Autodesk Fusion 360 part; units mm, degrees
note: some values were not read from the file. Chosen so that the rebuilt part matches the saved one: which bodies a step acts on.
(part 2 of 2)
extrude "Extrude1''''''''''''''''''''''''''''''" add sketch "Motor_Pulley_Sketch" along normal blind 6 from surface at 16 separate body makes body 36 in component "Motor_Pulley"
sketch "Tension_Slot_-11_16" plane through (0, 0, 0) normal (0, 0, 1) x (1, 0, 0) in component "Base_Plate_Al"
  line L0 (-12.7, 13) -> (-9.3, 13)
  line L1 (-9.3, 13) -> (-9.3, 19)
  line L2 (-9.3, 19) -> (-12.7, 19)
  line L3 (-12.7, 19) -> (-12.7, 13)
extrude "Extrude15'" cut sketch "Tension_Slot_-11_16" along normal blind 6 from surface at 1 bodies 1 in component "Base_Plate_Al"
sketch "Tension_Slot_11_16" plane through (0, 0, 0) normal (0, 0, 1) x (1, 0, 0) in component "Base_Plate_Al"
  line L0 (9.3, 13) -> (12.7, 13)
  line L1 (12.7, 13) -> (12.7, 19)
  line L2 (12.7, 19) -> (9.3, 19)
  line L3 (9.3, 19) -> (9.3, 13)
extrude "Extrude16" cut sketch "Tension_Slot_11_16" along normal blind 6 from surface at 1 bodies 1 in component "Base_Plate_Al"
sketch "Tension_Slot_-11_37" plane through (0, 0, 0) normal (0, 0, 1) x (1, 0, 0) in component "Base_Plate_Al"
  line L0 (-12.7, 34) -> (-9.3, 34)
  line L1 (-9.3, 34) -> (-9.3, 40)
  line L2 (-9.3, 40) -> (-12.7, 40)
  line L3 (-12.7, 40) -> (-12.7, 34)
extrude "Extrude17" cut sketch "Tension_Slot_-11_37" along normal blind 6 from surface at 1 bodies 1 in component "Base_Plate_Al"
sketch "Tension_Slot_11_37" plane through (0, 0, 0) normal (0, 0, 1) x (1, 0, 0) in component "Base_Plate_Al"
  line L0 (9.3, 34) -> (12.7, 34)
  line L1 (12.7, 34) -> (12.7, 40)
  line L2 (12.7, 40) -> (9.3, 40)
  line L3 (9.3, 40) -> (9.3, 34)
extrude "Extrude18" cut sketch "Tension_Slot_11_37" along normal blind 6 from surface at 1 bodies 1 in component "Base_Plate_Al"
sketch "Shaft_Bore" plane through (0, 0, 0) normal (1, 0, 0) x (0, 0, -1) in component "Weapon_Pulley"
  circle A0 centre (-38.5, 75) radius 2
extrude "Extrude2''''''''''''''''''''''''" cut sketch "Shaft_Bore" along normal mid plane 400 bodies 35 in component "Weapon_Pulley"
sketch "Shaft_Bore (2)" plane through (0, 0, 0) normal (1, 0, 0) x (0, 0, -1) in component "Left_Support"
  circle A0 centre (-38.5, 75) radius 2
extrude "Extrude2'''''''''''''''''''''''''" cut sketch "Shaft_Bore (2)" along normal mid plane 400 bodies 15 in component "Left_Support"
sketch "Shaft_Bore (3)" plane through (0, 0, 0) normal (1, 0, 0) x (0, 0, -1) in component "Right_Support"
  circle A0 centre (-38.5, 75) radius 2
extrude "Extrude2''''''''''''''''''''''''''" cut sketch "Shaft_Bore (3)" along normal mid plane 400 bodies 16 in component "Right_Support"
sketch "Shaft_Bore (4)" plane through (0, 0, 0) normal (1, 0, 0) x (0, 0, -1) in component "Motor_Pulley"
  circle A0 centre (-38.5, 25.75) radius 1.585
extrude "Extrude2'''''''''''''''''''''''''''" cut sketch "Shaft_Bore (4)" along normal mid plane 400 bodies 36 in component "Motor_Pulley"
sketch "Wedge_HoldDown_Clear" plane through (0, 0, 0) normal (0, 0, 1) x (1, 0, 0) in component "Front_Wedge_L"
  circle A0 centre (-73, 80) radius 1.7
  circle A1 centre (-50, 50) radius 1.7
extrude "Extrude5'''''''" cut sketch "Wedge_HoldDown_Clear" along normal blind 6 from surface at 4 bodies 12 in component "Front_Wedge_L"
sketch "Wedge_HoldDown_Clear (2)" plane through (0, 0, 0) normal (0, 0, 1) x (1, 0, 0) in component "Front_Wedge_R"
  circle A0 centre (50, 50) radius 1.7
  circle A1 centre (73, 80) radius 1.7
extrude "Extrude5''''''''" cut sketch "Wedge_HoldDown_Clear (2)" along normal blind 6 from surface at 4 bodies 13 in component "Front_Wedge_R"
sketch "ESC_Tekko32_Sketch" plane through (0, 0, 0) normal (0, 0, 1) x (1, 0, 0) in component "ESC_Tekko32"
  line L0 (17.85, 19.35) -> (52.15, 19.35)
  line L1 (52.15, 19.35) -> (52.15, 36.65)
  line L2 (52.15, 36.65) -> (17.85, 36.65)
  line L3 (17.85, 36.65) -> (17.85, 19.35)
extrude "Extrude1'''''''''''''''''''''''''''''''" add sketch "ESC_Tekko32_Sketch" along normal blind 4.5 from surface at 7 separate body makes body 37 in component "ESC_Tekko32"
sketch "Holder_ESC_Tekko32_Sketch" plane through (0, 0, 0) normal (0, 0, 1) x (1, 0, 0) in component "Holder_ESC_Tekko32"
  line L0 (16.05, 17.55) -> (53.95, 17.55)
  line L1 (53.95, 17.55) -> (53.95, 38.45)
  line L2 (53.95, 38.45) -> (16.05, 38.45)
  line L3 (16.05, 38.45) -> (16.05, 17.55)
extrude "Extrude1''''''''''''''''''''''''''''''''" add sketch "Holder_ESC_Tekko32_Sketch" along normal blind 5.5 from surface at 5 separate body makes body 38 in component "Holder_ESC_Tekko32"
sketch "Holder_ESC_Tekko32_Pocket" plane through (0, 0, 0) normal (0, 0, 1) x (1, 0, 0) in component "Holder_ESC_Tekko32"
  line L0 (17.65, 19.15) -> (52.35, 19.15)
  line L1 (52.35, 19.15) -> (52.35, 36.85)
  line L2 (52.35, 36.85) -> (17.65, 36.85)
  line L3 (17.65, 36.85) -> (17.65, 19.15)
extrude "Extrude2''''''''''''''''''''''''''''" cut sketch "Holder_ESC_Tekko32_Pocket" along normal blind 60 from surface at 7 bodies 38 in component "Holder_ESC_Tekko32"
sketch "Holder_ESC_Tekko32_TieGroove" plane through (0, 0, 0) normal (0, 0, 1) x (1, 0, 0) in component "Holder_ESC_Tekko32"
  line L0 (33, 16.55) -> (37, 16.55)
  line L1 (37, 16.55) -> (37, 39.45)
  line L2 (37, 39.45) -> (33, 39.45)
  line L3 (33, 39.45) -> (33, 16.55)
extrude "Extrude3''''''''''''''''" cut sketch "Holder_ESC_Tekko32_TieGroove" along normal blind 2.2 from surface at 4 bodies 38 in component "Holder_ESC_Tekko32"
sketch "Holder_ESC_Tekko32_FloorHoles" plane through (0, 0, 0) normal (0, 0, 1) x (1, 0, 0) in component "Holder_ESC_Tekko32"
  circle A0 centre (21.85, 28) radius 1.7
  circle A1 centre (48.15, 28) radius 1.7
extrude "Extrude4''''''''''''" cut sketch "Holder_ESC_Tekko32_FloorHoles" along normal blind 4 from surface at 4 bodies 38 in component "Holder_ESC_Tekko32"
sketch "Holder_ESC_Tekko32_PlateHoles" plane through (0, 0, 0) normal (0, 0, 1) x (1, 0, 0) in component "Base_Plate_Al"
  circle A0 centre (21.85, 28) radius 1.25
  circle A1 centre (48.15, 28) radius 1.25
extrude "Extrude23" cut sketch "Holder_ESC_Tekko32_PlateHoles" along normal blind 6 from surface at 1 bodies 1 in component "Base_Plate_Al"
sketch "Rx_ER6_Sketch" plane through (0, 0, 0) normal (0, 0, 1) x (1, 0, 0) in component "Rx_ER6"
  line L0 (-64.5, -84.5) -> (-39.5, -84.5)
  line L1 (-39.5, -84.5) -> (-39.5, -41.5)
  line L2 (-39.5, -41.5) -> (-64.5, -41.5)
  line L3 (-64.5, -41.5) -> (-64.5, -84.5)
extrude "Extrude1'''''''''''''''''''''''''''''''''" add sketch "Rx_ER6_Sketch" along normal blind 15 from surface at 7 separate body makes body 39 in component "Rx_ER6"
sketch "Holder_Rx_ER6_Sketch" plane through (0, 0, 0) normal (0, 0, 1) x (1, 0, 0) in component "Holder_Rx_ER6"
  line L0 (-66.3, -86.3) -> (-37.7, -86.3)
  line L1 (-37.7, -86.3) -> (-37.7, -39.7)
  line L2 (-37.7, -39.7) -> (-66.3, -39.7)
  line L3 (-66.3, -39.7) -> (-66.3, -86.3)
extrude "Extrude1''''''''''''''''''''''''''''''''''" add sketch "Holder_Rx_ER6_Sketch" along normal blind 16 from surface at 5 separate body makes body 40 in component "Holder_Rx_ER6"
sketch "Holder_Rx_ER6_Pocket" plane through (0, 0, 0) normal (0, 0, 1) x (1, 0, 0) in component "Holder_Rx_ER6"
  line L0 (-64.7, -84.7) -> (-39.3, -84.7)
  line L1 (-39.3, -84.7) -> (-39.3, -41.3)
  line L2 (-39.3, -41.3) -> (-64.7, -41.3)
  line L3 (-64.7, -41.3) -> (-64.7, -84.7)
extrude "Extrude2'''''''''''''''''''''''''''''" cut sketch "Holder_Rx_ER6_Pocket" along normal blind 60 from surface at 7 bodies 40 in component "Holder_Rx_ER6"
sketch "Holder_Rx_ER6_TieGroove" plane through (0, 0, 0) normal (0, 0, 1) x (1, 0, 0) in component "Holder_Rx_ER6"
  line L0 (-67.3, -65) -> (-36.7, -65)
  line L1 (-36.7, -65) -> (-36.7, -61)
  line L2 (-36.7, -61) -> (-67.3, -61)
  line L3 (-67.3, -61) -> (-67.3, -65)
extrude "Extrude3'''''''''''''''''" cut sketch "Holder_Rx_ER6_TieGroove" along normal blind 2.2 from surface at 4 bodies 40 in component "Holder_Rx_ER6"
sketch "Holder_Rx_ER6_FloorHoles" plane through (0, 0, 0) normal (0, 0, 1) x (1, 0, 0) in component "Holder_Rx_ER6"
  circle A0 centre (-52, -80.5) radius 1.7
  circle A1 centre (-52, -45.5) radius 1.7
extrude "Extrude4'''''''''''''" cut sketch "Holder_Rx_ER6_FloorHoles" along normal blind 4 from surface at 4 bodies 40 in component "Holder_Rx_ER6"
sketch "Holder_Rx_ER6_PlateHoles" plane through (0, 0, 0) normal (0, 0, 1) x (1, 0, 0) in component "Base_Plate_Al"
  circle A0 centre (-52, -80.5) radius 1.25
  circle A1 centre (-52, -45.5) radius 1.25
extrude "Extrude24" cut sketch "Holder_Rx_ER6_PlateHoles" along normal blind 6 from surface at 1 bodies 1 in component "Base_Plate_Al"
sketch "UBEC_5A_Sketch" plane through (0, 0, 0) normal (0, 0, 1) x (1, 0, 0) in component "UBEC_5A"
  line L0 (57.5, -76) -> (74.5, -76)
  line L1 (74.5, -76) -> (74.5, -26)
  line L2 (74.5, -26) -> (57.5, -26)
  line L3 (57.5, -26) -> (57.5, -76)
extrude "Extrude1'''''''''''''''''''''''''''''''''''" add sketch "UBEC_5A_Sketch" along normal blind 10 from surface at 7 separate body makes body 41 in component "UBEC_5A"
sketch "Holder_UBEC_5A_Sketch" plane through (0, 0, 0) normal (0, 0, 1) x (1, 0, 0) in component "Holder_UBEC_5A"
  line L0 (55.7, -77.8) -> (76.3, -77.8)
  line L1 (76.3, -77.8) -> (76.3, -24.2)
  line L2 (76.3, -24.2) -> (55.7, -24.2)
  line L3 (55.7, -24.2) -> (55.7, -77.8)
extrude "Extrude1''''''''''''''''''''''''''''''''''''" add sketch "Holder_UBEC_5A_Sketch" along normal blind 11 from surface at 5 separate body makes body 42 in component "Holder_UBEC_5A"
sketch "Holder_UBEC_5A_Pocket" plane through (0, 0, 0) normal (0, 0, 1) x (1, 0, 0) in component "Holder_UBEC_5A"
  line L0 (57.3, -76.2) -> (74.7, -76.2)
  line L1 (74.7, -76.2) -> (74.7, -25.8)
  line L2 (74.7, -25.8) -> (57.3, -25.8)
  line L3 (57.3, -25.8) -> (57.3, -76.2)
extrude "Extrude2''''''''''''''''''''''''''''''" cut sketch "Holder_UBEC_5A_Pocket" along normal blind 60 from surface at 7 bodies 42 in component "Holder_UBEC_5A"
sketch "Holder_UBEC_5A_TieGroove" plane through (0, 0, 0) normal (0, 0, 1) x (1, 0, 0) in component "Holder_UBEC_5A"
  line L0 (54.7, -53) -> (77.3, -53)
  line L1 (77.3, -53) -> (77.3, -49)
  line L2 (77.3, -49) -> (54.7, -49)
  line L3 (54.7, -49) -> (54.7, -53)
extrude "Extrude3''''''''''''''''''" cut sketch "Holder_UBEC_5A_TieGroove" along normal blind 2.2 from surface at 4 bodies 42 in component "Holder_UBEC_5A"
sketch "Holder_UBEC_5A_FloorHoles" plane through (0, 0, 0) normal (0, 0, 1) x (1, 0, 0) in component "Holder_UBEC_5A"
  circle A0 centre (66, -72) radius 1.7
  circle A1 centre (66, -30) radius 1.7
extrude "Extrude4''''''''''''''" cut sketch "Holder_UBEC_5A_FloorHoles" along normal blind 4 from surface at 4 bodies 42 in component "Holder_UBEC_5A"
sketch "Holder_UBEC_5A_PlateHoles" plane through (0, 0, 0) normal (0, 0, 1) x (1, 0, 0) in component "Base_Plate_Al"
  circle A0 centre (66, -72) radius 1.25
  circle A1 centre (66, -30) radius 1.25
extrude "Extrude25" cut sketch "Holder_UBEC_5A_PlateHoles" along normal blind 6 from surface at 1 bodies 1 in component "Base_Plate_Al"
sketch "DRV8874_A_Sketch" plane through (0, 0, 0) normal (0, 0, 1) x (1, 0, 0) in component "DRV8874_A"
  line L0 (-34.9, -81.6) -> (-17.1, -81.6)
  line L1 (-17.1, -81.6) -> (-17.1, -66.4)
  line L2 (-17.1, -66.4) -> (-34.9, -66.4)
  line L3 (-34.9, -66.4) -> (-34.9, -81.6)
extrude "Extrude1'''''''''''''''''''''''''''''''''''''" add sketch "DRV8874_A_Sketch" along normal blind 3 from surface at 7 separate body makes body 43 in component "DRV8874_A"
sketch "Holder_DRV8874_A_Sketch" plane through (0, 0, 0) normal (0, 0, 1) x (1, 0, 0) in component "Holder_DRV8874_A"
  line L0 (-36.7, -83.4) -> (-15.3, -83.4)
  line L1 (-15.3, -83.4) -> (-15.3, -64.6)
  line L2 (-15.3, -64.6) -> (-36.7, -64.6)
  line L3 (-36.7, -64.6) -> (-36.7, -83.4)
extrude "Extrude1''''''''''''''''''''''''''''''''''''''" add sketch "Holder_DRV8874_A_Sketch" along normal blind 4 from surface at 5 separate body makes body 44 in component "Holder_DRV8874_A"
sketch "Holder_DRV8874_A_Pocket" plane through (0, 0, 0) normal (0, 0, 1) x (1, 0, 0) in component "Holder_DRV8874_A"
  line L0 (-35.1, -81.8) -> (-16.9, -81.8)
  line L1 (-16.9, -81.8) -> (-16.9, -66.2)
  line L2 (-16.9, -66.2) -> (-35.1, -66.2)
  line L3 (-35.1, -66.2) -> (-35.1, -81.8)
extrude "Extrude2'''''''''''''''''''''''''''''''" cut sketch "Holder_DRV8874_A_Pocket" along normal blind 60 from surface at 7 bodies 44 in component "Holder_DRV8874_A"
sketch "Holder_DRV8874_A_TieGroove" plane through (0, 0, 0) normal (0, 0, 1) x (1, 0, 0) in component "Holder_DRV8874_A"
  line L0 (-28, -84.4) -> (-24, -84.4)
  line L1 (-24, -84.4) -> (-24, -63.6)
  line L2 (-24, -63.6) -> (-28, -63.6)
  line L3 (-28, -63.6) -> (-28, -84.4)
extrude "Extrude3'''''''''''''''''''" cut sketch "Holder_DRV8874_A_TieGroove" along normal blind 2.2 from surface at 4 bodies 44 in component "Holder_DRV8874_A"
sketch "Holder_DRV8874_A_FloorHoles" plane through (0, 0, 0) normal (0, 0, 1) x (1, 0, 0) in component "Holder_DRV8874_A"
  circle A0 centre (-31, -74) radius 1.7
  circle A1 centre (-21, -74) radius 1.7
extrude "Extrude4'''''''''''''''" cut sketch "Holder_DRV8874_A_FloorHoles" along normal blind 4 from surface at 4 bodies 44 in component "Holder_DRV8874_A"
sketch "Holder_DRV8874_A_PlateHoles" plane through (0, 0, 0) normal (0, 0, 1) x (1, 0, 0) in component "Base_Plate_Al"
  circle A0 centre (-31, -74) radius 1.25
  circle A1 centre (-21, -74) radius 1.25
extrude "Extrude26" cut sketch "Holder_DRV8874_A_PlateHoles" along normal blind 6 from surface at 1 bodies 1 in component "Base_Plate_Al"
sketch "DRV8874_B_Sketch" plane through (0, 0, 0) normal (0, 0, 1) x (1, 0, 0) in component "DRV8874_B"
  line L0 (-11.6, -83.9) -> (3.6, -83.9)
  line L1 (3.6, -83.9) -> (3.6, -66.1)
  line L2 (3.6, -66.1) -> (-11.6, -66.1)
  line L3 (-11.6, -66.1) -> (-11.6, -83.9)
extrude "Extrude1'''''''''''''''''''''''''''''''''''''''" add sketch "DRV8874_B_Sketch" along normal blind 3 from surface at 7 separate body makes body 45 in component "DRV8874_B"
sketch "Holder_DRV8874_B_Sketch" plane through (0, 0, 0) normal (0, 0, 1) x (1, 0, 0) in component "Holder_DRV8874_B"
  line L0 (-13.4, -85.7) -> (5.4, -85.7)
  line L1 (5.4, -85.7) -> (5.4, -64.3)
  line L2 (5.4, -64.3) -> (-13.4, -64.3)
  line L3 (-13.4, -64.3) -> (-13.4, -85.7)
extrude "Extrude1''''''''''''''''''''''''''''''''''''''''" add sketch "Holder_DRV8874_B_Sketch" along normal blind 4 from surface at 5 separate body makes body 46 in component "Holder_DRV8874_B"
sketch "Holder_DRV8874_B_Pocket" plane through (0, 0, 0) normal (0, 0, 1) x (1, 0, 0) in component "Holder_DRV8874_B"
  line L0 (-11.8, -84.1) -> (3.8, -84.1)
  line L1 (3.8, -84.1) -> (3.8, -65.9)
  line L2 (3.8, -65.9) -> (-11.8, -65.9)
  line L3 (-11.8, -65.9) -> (-11.8, -84.1)
extrude "Extrude2''''''''''''''''''''''''''''''''" cut sketch "Holder_DRV8874_B_Pocket" along normal blind 60 from surface at 7 bodies 46 in component "Holder_DRV8874_B"
sketch "Holder_DRV8874_B_TieGroove" plane through (0, 0, 0) normal (0, 0, 1) x (1, 0, 0) in component "Holder_DRV8874_B"
  line L0 (-14.4, -77) -> (6.4, -77)
  line L1 (6.4, -77) -> (6.4, -73)
  line L2 (6.4, -73) -> (-14.4, -73)
  line L3 (-14.4, -73) -> (-14.4, -77)
extrude "Extrude3''''''''''''''''''''" cut sketch "Holder_DRV8874_B_TieGroove" along normal blind 2.2 from surface at 4 bodies 46 in component "Holder_DRV8874_B"
sketch "Holder_DRV8874_B_FloorHoles" plane through (0, 0, 0) normal (0, 0, 1) x (1, 0, 0) in component "Holder_DRV8874_B"
  circle A0 centre (-4, -80) radius 1.7
  circle A1 centre (-4, -70) radius 1.7
extrude "Extrude4''''''''''''''''" cut sketch "Holder_DRV8874_B_FloorHoles" along normal blind 4 from surface at 4 bodies 46 in component "Holder_DRV8874_B"
sketch "Holder_DRV8874_B_PlateHoles" plane through (0, 0, 0) normal (0, 0, 1) x (1, 0, 0) in component "Base_Plate_Al"
  circle A0 centre (-4, -80) radius 1.25
  circle A1 centre (-4, -70) radius 1.25
extrude "Extrude27" cut sketch "Holder_DRV8874_B_PlateHoles" along normal blind 6 from surface at 1 bodies 1 in component "Base_Plate_Al"
sketch "ESP32_DevKit_Sketch" plane through (0, 0, 0) normal (0, 0, 1) x (1, 0, 0) in component "ESP32_DevKit"
  line L0 (-25.75, -52.15) -> (25.75, -52.15)
  line L1 (25.75, -52.15) -> (25.75, -23.85)
  line L2 (25.75, -23.85) -> (-25.75, -23.85)
  line L3 (-25.75, -23.85) -> (-25.75, -52.15)
extrude "Extrude1'''''''''''''''''''''''''''''''''''''''''" add sketch "ESP32_DevKit_Sketch" along normal blind 1.6 from surface at 25 separate body makes body 47 in component "ESP32_DevKit"
sketch "ESP32_Holes" plane through (0, 0, 0) normal (0, 0, 1) x (1, 0, 0) in component "ESP32_DevKit"
  circle A0 centre (-23.6, -49.7) radius 1.3
  circle A1 centre (-23.6, -26.3) radius 1.3
  circle A2 centre (23.6, -49.7) radius 1.3
  circle A3 centre (23.6, -26.3) radius 1.3
extrude "Extrude2'''''''''''''''''''''''''''''''''" cut sketch "ESP32_Holes" along normal blind 3.6 from surface at 24 bodies 47 in component "ESP32_DevKit"
sketch "ESP32_Module_Sketch" plane through (0, 0, 0) normal (0, 0, 1) x (1, 0, 0) in component "ESP32_DevKit"
  line L0 (-25.75, -47) -> (-0.25, -47)
  line L1 (-0.25, -47) -> (-0.25, -29)
  line L2 (-0.25, -29) -> (-25.75, -29)
  line L3 (-25.75, -29) -> (-25.75, -47)
extrude "Extrude3'''''''''''''''''''''" add sketch "ESP32_Module_Sketch" along normal blind 3.1 from surface at 26.6 separate body makes body 48 in component "ESP32_DevKit"
sketch "ESP32_Dupont_Keepout_A_Sketch" plane through (0, 0, 0) normal (0, 0, 1) x (1, 0, 0) in component "ESP32_DevKit"
  line L0 (-20.72, -51.97) -> (14.88, -51.97)
  line L1 (14.88, -51.97) -> (14.88, -49.43)
  line L2 (14.88, -49.43) -> (-20.72, -49.43)
  line L3 (-20.72, -49.43) -> (-20.72, -51.97)
extrude "Extrude4'''''''''''''''''" add sketch "ESP32_Dupont_Keepout_A_Sketch" along normal blind 16.5 from surface at 8.5 separate body makes body 49 in component "ESP32_DevKit"
sketch "ESP32_Dupont_Keepout_B_Sketch" plane through (0, 0, 0) normal (0, 0, 1) x (1, 0, 0) in component "ESP32_DevKit"
  line L0 (-20.72, -26.57) -> (14.88, -26.57)
  line L1 (14.88, -26.57) -> (14.88, -24.03)
  line L2 (14.88, -24.03) -> (-20.72, -24.03)
  line L3 (-20.72, -24.03) -> (-20.72, -26.57)
extrude "Extrude5'''''''''" add sketch "ESP32_Dupont_Keepout_B_Sketch" along normal blind 16.5 from surface at 8.5 separate body makes body 50 in component "ESP32_DevKit"
sketch "Holder_ESP32_Sketch" plane through (0, 0, 0) normal (0, 0, 1) x (1, 0, 0) in component "Holder_ESP32"
  line L0 (-27.75, -54.15) -> (27.75, -54.15)
  line L1 (27.75, -54.15) -> (27.75, -21.85)
  line L2 (27.75, -21.85) -> (-27.75, -21.85)
  line L3 (-27.75, -21.85) -> (-27.75, -54.15)
extrude "Extrude1''''''''''''''''''''''''''''''''''''''''''" add sketch "Holder_ESP32_Sketch" along normal blind 2 from surface at 5 separate body makes body 51 in component "Holder_ESP32"
sketch "Holder_ESP32_Posts" plane through (0, 0, 0) normal (0, 0, 1) x (1, 0, 0) in component "Holder_ESP32"
  circle A0 centre (-23.6, -49.7) radius 2.25
  circle A1 centre (-23.6, -26.3) radius 2.25
  circle A2 centre (23.6, -49.7) radius 2.25
  circle A3 centre (23.6, -26.3) radius 2.25
extrude "Extrude2''''''''''''''''''''''''''''''''''" add sketch "Holder_ESP32_Posts" along normal blind 18 from surface at 7 bodies 51 in component "Holder_ESP32"
sketch "Holder_ESP32_Window" plane through (0, 0, 0) normal (0, 0, 1) x (1, 0, 0) in component "Holder_ESP32"
  line L0 (-9, -47.15) -> (9, -47.15)
  line L1 (9, -47.15) -> (9, -28.85)
  line L2 (9, -28.85) -> (-9, -28.85)
  line L3 (-9, -28.85) -> (-9, -47.15)
extrude "Extrude3''''''''''''''''''''''" cut sketch "Holder_ESP32_Window" along normal blind 4 from surface at 4 bodies 51 in component "Holder_ESP32"
sketch "Holder_ESP32_PostPilots" plane through (0, 0, 0) normal (0, 0, 1) x (1, 0, 0) in component "Holder_ESP32"
  circle A0 centre (-23.6, -49.7) radius 0.8
  circle A1 centre (-23.6, -26.3) radius 0.8
  circle A2 centre (23.6, -49.7) radius 0.8
  circle A3 centre (23.6, -26.3) radius 0.8
extrude "Extrude4''''''''''''''''''" cut sketch "Holder_ESP32_PostPilots" against normal blind 8 from surface at 25 bodies 51 in component "Holder_ESP32"
sketch "Holder_ESP32_Screws" plane through (0, 0, 0) normal (0, 0, 1) x (1, 0, 0) in component "Holder_ESP32"
  circle A0 centre (-15, -38) radius 1.7
  circle A1 centre (15, -38) radius 1.7
extrude "Extrude5''''''''''" cut sketch "Holder_ESP32_Screws" along normal blind 4 from surface at 4 bodies 51 in component "Holder_ESP32"
sketch "Holder_ESP32_PlateHoles" plane through (0, 0, 0) normal (0, 0, 1) x (1, 0, 0) in component "Base_Plate_Al"
  circle A0 centre (-15, -38) radius 1.25
  circle A1 centre (15, -38) radius 1.25
extrude "Extrude28" cut sketch "Holder_ESP32_PlateHoles" along normal blind 6 from surface at 1 bodies 1 in component "Base_Plate_Al"
sketch "DXF_Base_Plate_Al" plane through (0, 0, 3) normal (0, 0, -1) x (-1, 0, 0) in component "Base_Plate_Al"
  circle A0 centre (4, -80) radius 1.25
  circle A1 centre (4, -70) radius 1.25
  circle A2 centre (-66, -72) radius 1.25
  circle A3 centre (-66, -30) radius 1.25
  circle A4 centre (-21.85, 28) radius 1.25
  circle A5 centre (-48.15, 28) radius 1.25
  line L0 (12.7, 40) -> (12.7, 34)
  line L1 (12.7, 34) -> (9.3, 34)
  line L2 (9.3, 34) -> (9.3, 40)
  line L3 (9.3, 40) -> (12.7, 40)
  line L4 (12.7, 19) -> (12.7, 13)
  line L5 (12.7, 13) -> (9.3, 13)
  line L6 (9.3, 13) -> (9.3, 19)
  line L7 (9.3, 19) -> (12.7, 19)
  circle A6 centre (34, -46) radius 1.45
  circle A7 centre (-34, -30) radius 1.45
  circle A8 centre (34, -30) radius 1.45
  circle A9 centre (-34, -46) radius 1.45
  circle A10 centre (38.7, -14) radius 1.7
  circle A11 centre (51, 14) radius 1.7
  circle A12 centre (51, -14) radius 1.7
  circle A13 centre (38.7, 14) radius 1.7
  circle A14 centre (-73, 80) radius 1.7
  circle A15 centre (-50, 50) radius 1.7
  circle A16 centre (73, 80) radius 1.7
  circle A17 centre (50, 50) radius 1.7
  circle A18 centre (75, 35) radius 1.7
  circle A19 centre (-75, -85) radius 1.7
  circle A20 centre (75, -85) radius 1.7
  circle A21 centre (-75, 35) radius 1.7
  line L8 (-80, 24) -> (-58, 24)
  line L9 (-58, 24) -> (-58, -24)
  line L10 (-58, -24) -> (-80, -24)
  line L11 (-80, -24) -> (-80, -90)
  line L12 (-80, -90) -> (80, -90)
  line L13 (80, -90) -> (80, -24)
  line L14 (80, -24) -> (58, -24)
  line L15 (58, -24) -> (58, 24)
  line L16 (58, 24) -> (80, 24)
  line L17 (80, 24) -> (80, 90)
  line L18 (80, 90) -> (-80, 90)
  line L19 (-80, 90) -> (-80, 24)
  circle A22 centre (-51, 14) radius 1.7
  circle A23 centre (-38.7, -14) radius 1.7
  circle A24 centre (-38.7, 14) radius 1.7
  circle A25 centre (-51, -14) radius 1.7
  circle A26 centre (-51.5, -70) radius 1.45
  circle A27 centre (-32.5, -70) radius 1.45
  line L20 (-9.3, 19) -> (-9.3, 13)
  line L21 (-9.3, 13) -> (-12.7, 13)
  line L22 (-12.7, 13) -> (-12.7, 19)
  line L23 (-12.7, 19) -> (-9.3, 19)
  line L24 (-9.3, 40) -> (-9.3, 34)
  line L25 (-9.3, 34) -> (-12.7, 34)
  line L26 (-12.7, 34) -> (-12.7, 40)
  line L27 (-12.7, 40) -> (-9.3, 40)
  circle A28 centre (52, -45.5) radius 1.25
  circle A29 centre (52, -80.5) radius 1.25
  circle A30 centre (21, -74) radius 1.25
  circle A31 centre (31, -74) radius 1.25
  circle A32 centre (-15, -38) radius 1.25
  circle A33 centre (15, -38) radius 1.25
sketch "DXF_Left_Side_Plate_Al" plane through (-78, 0, 0) normal (1, 0, 0) x (0, 0, -1) in component "Left_Side_Plate_Al"
  circle A0 centre (-44, -85) radius 1.7
  circle A1 centre (-44, 35) radius 1.7
  line L0 (-5, -26) -> (-47, -26)
  line L1 (-47, -26) -> (-47, 26)
  line L2 (-47, 26) -> (-5, 26)
  line L3 (-5, 26) -> (-5, 40)
  line L4 (-5, 40) -> (-83, 40)
  line L5 (-83, 40) -> (-83, -90)
  line L6 (-83, -90) -> (-5, -90)
  line L7 (-5, -90) -> (-5, -26)
sketch "DXF_Right_Side_Plate_Al" plane through (78, 0, 0) normal (-1, 0, 0) x (0, 0, 1) in component "Right_Side_Plate_Al"
  circle A0 centre (44, -85) radius 1.7
  circle A1 centre (44, 35) radius 1.7
  line L0 (5, 26) -> (47, 26)
  line L1 (47, 26) -> (47, -26)
  line L2 (47, -26) -> (5, -26)
  line L3 (5, -26) -> (5, -90)
  line L4 (5, -90) -> (83, -90)
  line L5 (83, -90) -> (83, 40)
  line L6 (83, 40) -> (5, 40)
  line L7 (5, 40) -> (5, 26)
sketch "DXF_Front_Wedge_L" plane through (-80, 0, 0) normal (-1, 0, 0) x (0, 0, 1) in component "Front_Wedge_L"
  line L0 (5, 40) -> (83, 40)
  line L1 (83, 40) -> (5, 90)
  line L2 (5, 90) -> (5, 40)
sketch "DXF_Front_Wedge_R" plane through (80, 0, 0) normal (1, 0, 0) x (0, 0, -1) in component "Front_Wedge_R"
  line L0 (-83, 40) -> (-5, 40)
  line L1 (-5, 40) -> (-5, 90)
  line L2 (-5, 90) -> (-83, 40)
sketch "FingerTech_Switch_Adapter_Outline" plane through (0, 0, 0) normal (0, 0, 1) x (1, 0, 0) in component "FingerTech_Switch_Adapter"
  line L0 (28, -79) -> (56, -79)
  line L1 (56, -79) -> (56, -61)
  line L2 (56, -61) -> (28, -61)
  line L3 (28, -61) -> (28, -79)
extrude "Extrude1'''''''''''''''''''''''''''''''''''''''''''" add sketch "FingerTech_Switch_Adapter_Outline" along normal blind 4 from surface at 45 separate body makes body 52 in component "FingerTech_Switch_Adapter"
sketch "Adapter_Post_Clearance_M3" plane through (0, 0, 0) normal (0, 0, 1) x (1, 0, 0) in component "FingerTech_Switch_Adapter"
  circle A0 centre (32.5, -70) radius 1.7
  circle A1 centre (51.5, -70) radius 1.7
extrude "Extrude2'''''''''''''''''''''''''''''''''''" cut sketch "Adapter_Post_Clearance_M3" along normal blind 6 from surface at 44 bodies 52 in component "FingerTech_Switch_Adapter"
sketch "Adapter_Switch_Clearance_M2" plane through (0, 0, 0) normal (0, 0, 1) x (1, 0, 0) in component "FingerTech_Switch_Adapter"
  circle A0 centre (38.19, -70) radius 1.1
  circle A1 centre (45.81, -70) radius 1.1
extrude "Extrude3'''''''''''''''''''''''" cut sketch "Adapter_Switch_Clearance_M2" along normal blind 6 from surface at 44 bodies 52 in component "FingerTech_Switch_Adapter"
sketch "FingerTech_Mini_Switch_Envelope_Outline" plane through (0, 0, 0) normal (0, 0, 1) x (1, 0, 0) in component "FingerTech_Mini_Switch_Envelope"
  line L0 (35.65, -76.35) -> (48.35, -76.35)
  line L1 (48.35, -76.35) -> (48.35, -63.65)
  line L2 (48.35, -63.65) -> (35.65, -63.65)
  line L3 (35.65, -63.65) -> (35.65, -76.35)
extrude "Extrude1''''''''''''''''''''''''''''''''''''''''''''" add sketch "FingerTech_Mini_Switch_Envelope_Outline" along normal blind 6.35 from surface at 49 separate body makes body 53 in component "FingerTech_Mini_Switch_Envelope"
sketch "FingerTech_Mount_Holes_M2" plane through (0, 0, 0) normal (0, 0, 1) x (1, 0, 0) in component "FingerTech_Mini_Switch_Envelope"
  circle A0 centre (38.19, -70) radius 1
  circle A1 centre (45.81, -70) radius 1
extrude "Extrude2''''''''''''''''''''''''''''''''''''" cut sketch "FingerTech_Mount_Holes_M2" along normal blind 9 from surface at 48 bodies 53 in component "FingerTech_Mini_Switch_Envelope"
sketch "FingerTech_Access_Patch" plane through (0, 0, 0) normal (0, 0, 1) x (1, 0, 0) in component "Top_Cover"
  line L0 (31, -79) -> (53, -79)
  line L1 (53, -79) -> (53, -61)
  line L2 (53, -61) -> (31, -61)
  line L3 (31, -61) -> (31, -79)
extrude "Extrude7''''" add sketch "FingerTech_Access_Patch" along normal blind 2 from surface at 83 bodies 6 in component "Top_Cover"
sketch "FingerTech_Hex_Access_6mm" plane through (0, 0, 0) normal (0, 0, 1) x (1, 0, 0) in component "Top_Cover"
  circle A0 centre (42, -70) radius 3
extrude "Extrude8''" cut sketch "FingerTech_Hex_Access_6mm" along normal blind 4 from surface at 82 bodies 6 in component "Top_Cover"
sketch "Beater_Outer_65x20" plane through (0, 0, 0) normal (0, 0, 1) x (1, 0, 0) in component "Beater_Rotor_Concept"
  line L0 (-20, 42.5) -> (14, 42.5)
  line L1 (14, 42.5) -> (14, 107.5)
  line L2 (14, 107.5) -> (-20, 107.5)
  line L3 (-20, 107.5) -> (-20, 42.5)
extrude "Extrude1'''''''''''''''''''''''''''''''''''''''''''''" add sketch "Beater_Outer_65x20" along normal blind 20 from surface at 28.5 separate body makes body 54 in component "Beater_Rotor_Concept"
sketch "Beater_Through_Window" plane through (0, 0, 0) normal (0, 0, 1) x (1, 0, 0) in component "Beater_Rotor_Concept"
  line L0 (-16, 52.5) -> (10, 52.5)
  line L1 (10, 52.5) -> (10, 97.5)
  line L2 (10, 97.5) -> (-16, 97.5)
  line L3 (-16, 97.5) -> (-16, 52.5)
extrude "Extrude2'''''''''''''''''''''''''''''''''''''" cut sketch "Beater_Through_Window" along normal blind 21 from surface at 28 bodies 54 in component "Beater_Rotor_Concept"
sketch "Beater_Shaft_Bore_4mm_Provisional" plane through (0, 0, 0) normal (1, 0, 0) x (0, 0, -1) in component "Beater_Rotor_Concept"
  circle A0 centre (-38.5, 75) radius 2
extrude "Extrude3''''''''''''''''''''''''" cut sketch "Beater_Shaft_Bore_4mm_Provisional" along normal mid plane 80 bodies 54 in component "Beater_Rotor_Concept"
sketch "Beater_Rotation_Radius_32p5" plane through (0, 0, 0) normal (1, 0, 0) x (0, 0, -1) in component "Beater_Sweep_Envelope"
  circle A0 centre (-38.5, 75) radius 32.5
extrude "Extrude1''''''''''''''''''''''''''''''''''''''''''''''" add sketch "Beater_Rotation_Radius_32p5" along normal blind 34 from surface at -20 separate body makes body 55 in component "Beater_Sweep_Envelope"
component "01_Chassis" placed x (1, 0, 0) y (0, 1, 0) z (0, 0, 1) at (0, 0, 0)
component "02_Drivetrain" placed x (1, 0, 0) y (0, 1, 0) z (0, 0, 1) at (0, 0, 0)
component "03_Front_Spinner" placed x (1, 0, 0) y (0, 1, 0) z (0, 0, 1) at (0, 0, 0)
component "05_Electronics" placed x (1, 0, 0) y (0, 1, 0) z (0, 0, 1) at (0, 0, 0)
component "06_3D_Printed" placed x (1, 0, 0) y (0, 1, 0) z (0, 0, 1) at (0, 0, 0)
component "Base_Plate_Al" placed x (1, 0, 0) y (0, 1, 0) z (0, 0, 1) at (0, 0, 0) in component "01_Chassis"
component "Left_Side_Plate_Al" placed x (1, 0, 0) y (0, 1, 0) z (0, 0, 1) at (0, 0, 0) in component "01_Chassis"
component "Right_Side_Plate_Al" placed x (1, 0, 0) y (0, 1, 0) z (0, 0, 1) at (0, 0, 0) in component "01_Chassis"
component "Top_Cover" placed x (1, 0, 0) y (0, 1, 0) z (0, 0, 1) at (0, 0, 0) in component "01_Chassis"
component "Front_Wedge_L" placed x (1, 0, 0) y (0, 1, 0) z (0, 0, 1) at (0, 0, 0) in component "01_Chassis"
component "Front_Wedge_R" placed x (1, 0, 0) y (0, 1, 0) z (0, 0, 1) at (0, 0, 0) in component "01_Chassis"
component "Standoffs_Fasteners" placed x (1, 0, 0) y (0, 1, 0) z (0, 0, 1) at (0, 0, 0) in component "01_Chassis"
component "Left_Wheel" placed x (1, 0, 0) y (0, 1, 0) z (0, 0, 1) at (0, 0, 0) in component "02_Drivetrain"
component "Right_Wheel" placed x (1, 0, 0) y (0, 1, 0) z (0, 0, 1) at (0, 0, 0) in component "02_Drivetrain"
component "TT_Gearbox_L" placed x (1, 0, 0) y (0, 1, 0) z (0, 0, 1) at (0, 0, 0) in component "02_Drivetrain"
component "TT_Motor_Can_L" placed x (1, 0, 0) y (0, 1, 0) z (0, 0, 1) at (0, 0, 0) in component "02_Drivetrain"
component "TT_Gearbox_R" placed x (1, 0, 0) y (0, 1, 0) z (0, 0, 1) at (0, 0, 0) in component "02_Drivetrain"
component "TT_Motor_Can_R" placed x (1, 0, 0) y (0, 1, 0) z (0, 0, 1) at (0, 0, 0) in component "02_Drivetrain"
component "TT_Motor_Mount_L" placed x (1, 0, 0) y (0, 1, 0) z (0, 0, 1) at (0, 0, 0) in component "02_Drivetrain"
component "TT_Motor_Clamp_L" placed x (1, 0, 0) y (0, 1, 0) z (0, 0, 1) at (0, 0, 0) in component "02_Drivetrain"
component "TT_Motor_Mount_R" placed x (1, 0, 0) y (0, 1, 0) z (0, 0, 1) at (0, 0, 0) in component "02_Drivetrain"
component "TT_Motor_Clamp_R" placed x (1, 0, 0) y (0, 1, 0) z (0, 0, 1) at (0, 0, 0) in component "02_Drivetrain"
component "Spinner_Shaft" placed x (1, 0, 0) y (0, 1, 0) z (0, 0, 1) at (0, 0, 0) in component "03_Front_Spinner"
component "Left_Support" placed x (1, 0, 0) y (0, 1, 0) z (0, 0, 1) at (0, 0, 0) in component "03_Front_Spinner"
component "Right_Support" placed x (1, 0, 0) y (0, 1, 0) z (0, 0, 1) at (0, 0, 0) in component "03_Front_Spinner"
component "Spinner_Motor" placed x (1, 0, 0) y (0, 1, 0) z (0, 0, 1) at (0, 0, 0) in component "03_Front_Spinner"
component "Spinner_Motor_Cradle" placed x (1, 0, 0) y (0, 1, 0) z (0, 0, 1) at (0, 0, 0) in component "03_Front_Spinner"
component "Weapon_Pulley" placed x (1, 0, 0) y (0, 1, 0) z (0, 0, 1) at (0, 0, 0) in component "03_Front_Spinner"
component "Motor_Pulley" placed x (1, 0, 0) y (0, 1, 0) z (0, 0, 1) at (0, 0, 0) in component "03_Front_Spinner"
component "ESC_Tekko32" placed x (1, 0, 0) y (0, 1, 0) z (0, 0, 1) at (0, 0, 0) in component "03_Front_Spinner"
component "Beater_Rotor_Concept" placed x (1, 0, 0) y (0, 1, 0) z (0, 0, 1) at (0, 0, 0) in component "03_Front_Spinner"
component "Beater_Sweep_Envelope" placed x (1, 0, 0) y (0, 1, 0) z (0, 0, 1) at (0, 0, 0) in component "03_Front_Spinner"
component "Cable_Routing_Keepouts" placed x (1, 0, 0) y (0, 1, 0) z (0, 0, 1) at (0, 0, 0) in component "05_Electronics"
component "Battery_and_Tray" placed x (1, 0, 0) y (0, 1, 0) z (0, 0, 1) at (0, 0, 0) in component "05_Electronics"
component "Rx_ER6" placed x (1, 0, 0) y (0, 1, 0) z (0, 0, 1) at (0, 0, 0) in component "05_Electronics"
component "UBEC_5A" placed x (1, 0, 0) y (0, 1, 0) z (0, 0, 1) at (0, 0, 0) in component "05_Electronics"
component "DRV8874_A" placed x (1, 0, 0) y (0, 1, 0) z (0, 0, 1) at (0, 0, 0) in component "05_Electronics"
component "DRV8874_B" placed x (1, 0, 0) y (0, 1, 0) z (0, 0, 1) at (0, 0, 0) in component "05_Electronics"
component "ESP32_DevKit" placed x (1, 0, 0) y (0, 1, 0) z (0, 0, 1) at (0, 0, 0) in component "05_Electronics"
component "FingerTech_Mini_Switch_Envelope" placed x (1, 0, 0) y (0, 1, 0) z (0, 0, 1) at (0, 0, 0) in component "05_Electronics"
component "Wire_Clips" placed x (1, 0, 0) y (0, 1, 0) z (0, 0, 1) at (0, 0, 0) in component "06_3D_Printed"
component "Non_Structural_Covers" placed x (1, 0, 0) y (0, 1, 0) z (0, 0, 1) at (0, 0, 0) in component "06_3D_Printed"
component "TPU_Bumpers" placed x (1, 0, 0) y (0, 1, 0) z (0, 0, 1) at (0, 0, 0) in component "06_3D_Printed"
component "Battery_Holder" placed x (1, 0, 0) y (0, 1, 0) z (0, 0, 1) at (0, 0, 0) in component "06_3D_Printed"
component "Batt_Post_1" placed x (1, 0, 0) y (0, 1, 0) z (0, 0, 1) at (0, 0, 0) in component "06_3D_Printed"
component "Batt_Post_2" placed x (1, 0, 0) y (0, 1, 0) z (0, 0, 1) at (0, 0, 0) in component "06_3D_Printed"
component "Batt_Post_3" placed x (1, 0, 0) y (0, 1, 0) z (0, 0, 1) at (0, 0, 0) in component "06_3D_Printed"
component "Batt_Post_4" placed x (1, 0, 0) y (0, 1, 0) z (0, 0, 1) at (0, 0, 0) in component "06_3D_Printed"
component "Disconnect_Post_1" placed x (1, 0, 0) y (0, 1, 0) z (0, 0, 1) at (0, 0, 0) in component "06_3D_Printed"
component "Disconnect_Post_2" placed x (1, 0, 0) y (0, 1, 0) z (0, 0, 1) at (0, 0, 0) in component "06_3D_Printed"
component "Holder_ESC_Tekko32" placed x (1, 0, 0) y (0, 1, 0) z (0, 0, 1) at (0, 0, 0) in component "06_3D_Printed"
component "Holder_Rx_ER6" placed x (1, 0, 0) y (0, 1, 0) z (0, 0, 1) at (0, 0, 0) in component "06_3D_Printed"
component "Holder_UBEC_5A" placed x (1, 0, 0) y (0, 1, 0) z (0, 0, 1) at (0, 0, 0) in component "06_3D_Printed"
component "Holder_DRV8874_A" placed x (1, 0, 0) y (0, 1, 0) z (0, 0, 1) at (0, 0, 0) in component "06_3D_Printed"
component "Holder_DRV8874_B" placed x (1, 0, 0) y (0, 1, 0) z (0, 0, 1) at (0, 0, 0) in component "06_3D_Printed"
component "Holder_ESP32" placed x (1, 0, 0) y (0, 1, 0) z (0, 0, 1) at (0, 0, 0) in component "06_3D_Printed"
component "FingerTech_Switch_Adapter" placed x (1, 0, 0) y (0, 1, 0) z (0, 0, 1) at (0, 0, 0) in component "06_3D_Printed"
component "Rear_Panel" placed x (1, 0, 0) y (0, 1, 0) z (0, 0, 1) at (0, 0, 0) in component "Non_Structural_Covers"
component "06_3D_Printed" placed x (1, 0, 0) y (0, 1, 0) z (0, 0, 1) at (0, 0, 0) in component "TPU_Bumpers"
equation "body_L = 180 mm" comment "Body length"
equation "body_W = 160 mm" comment "Body width incl. wheels"
equation "body_H = 80 mm" comment "Chassis height - raised from 70mm to give spinner sweep safe clearance under top cover"
equation "base_t = 2 mm" comment "DECIDED 2026-09-23: 2 mm aluminium plate (user approved)"
equation "side_t = 2 mm" comment "DECIDED 2026-09-23: 2 mm aluminium plate (user approved)"
equation "ground_clearance = 3 mm" comment "Ground clearance target"
equation "wheel_OD = 42 mm" comment "CONFIRMED: 42mm TT-motor wheel"
equation "wheel_W = 19 mm" comment "CONFIRMED (typical TT wheel width; verify against actual supplier spec)"
equation "motor_OD = 25 mm" comment "Gear motor housing envelope"
equation "pcb_L = 60 mm" comment "Control PCB placeholder length"
equation "pcb_W = 50 mm" comment "Control PCB placeholder width"
equation "pcb_keepout_H = 22 mm" comment "PCB top keepout height (placeholder)"
equation "assembly_clearance = 1 mm" comment "Generic assembly clearance"
equation "d14 = body_W"
equation "d15 = body_L"
equation "d16 = wheel_W"
equation "d17 = wheel_OD"
equation "d18 = wheel_W"
equation "d19 = wheel_OD"
equation "d20 = pcb_W"
equation "d21 = pcb_L"
equation "d26 = body_W"
equation "d27 = body_L"
equation "d28 = -base_t"
equation "d56 = -body_W / 2"
equation "d58 = body_H - base_t"
equation "d59 = body_L"
equation "d60 = side_t"
equation "d62 = body_W / 2"
equation "d64 = body_H - base_t"
equation "d65 = body_L"
equation "d66 = -side_t"
equation "d68 = -body_W / 2"
equation "d70 = wheel_OD"
equation "d71 = wheel_W"
equation "d73 = body_W / 2"
equation "d75 = wheel_OD"
equation "d76 = -wheel_W"
equation "spinner_gap_W = 70 mm" comment "MOCK layout gap for front spinner - NOT_FOR_MANUFACTURING, confirm with real weapon assembly"
equation "wedge_depth = 50 mm" comment "MOCK front wedge depth (front-to-back) - NOT_FOR_MANUFACTURING placeholder"
equation "d104 = body_H - base_t"
equation "d106 = body_W"
equation "d107 = body_L"
equation "d108 = base_t"
equation "battery_mock_L = 104 mm" comment "CONFIRMED: 3S 2200mAh LiPo typical size (Turnigy/GNB-class, ~500-700 THB Thai retail)"
equation "battery_mock_W = 35 mm" comment "MOCK 3S LiPo envelope width - NOT_FOR_MANUFACTURING"
equation "battery_mock_H = 27 mm" comment "MOCK 3S LiPo envelope height - NOT_FOR_MANUFACTURING"
equation "pcb_t = 1.6 mm" comment "Standard PCB thickness placeholder"
equation "module_mock_L = 25 mm" comment "MOCK small electronics module envelope length (driver/BEC/receiver/disconnect) - NOT_FOR_MANUFACTURING"
equation "module_mock_W = 20 mm" comment "MOCK small electronics module envelope width - NOT_FOR_MANUFACTURING"
equation "module_mock_H = 10 mm" comment "MOCK small electronics module envelope height - NOT_FOR_MANUFACTURING"
equation "tt_gearbox_L = 24 mm" comment "TT motor gearbox length along shaft axis - TYPICAL VALUE, confirm exact supplier datasheet before drilling mount holes"
equation "tt_gearbox_W = 22 mm" comment "TT motor gearbox cross-section width - TYPICAL VALUE, confirm before mount holes"
equation "tt_gearbox_H = 18 mm" comment "TT motor gearbox cross-section height - TYPICAL VALUE, confirm before mount holes"
equation "tt_can_D = 20 mm" comment "TT motor can (motor body) diameter - TYPICAL VALUE"
equation "tt_can_L = 25 mm" comment "TT motor can (motor body) length - TYPICAL VALUE"
equation "tt_shaft_D = 5 mm" comment "TT motor output D-shaft diameter - TYPICAL VALUE, confirm before hub fit"
equation "tt_shaft_L = 10 mm" comment "TT motor output shaft protrusion length - TYPICAL VALUE"
equation "d208 = wheel_OD / 2"
equation "d209 = wheel_OD / 2"
equation "d218 = side_t * 5"
equation "d220 = side_t * 5"
equation "d222 = side_t * 5"
equation "d224 = side_t * 5"
equation "d226 = -body_W / 2 + wheel_W"
equation "d228 = tt_gearbox_H"
equation "d229 = tt_gearbox_W"
equation "d230 = tt_gearbox_L"
equation "d234 = tt_can_D"
equation "d237 = -tt_can_L"
equation "d239 = body_W / 2 - wheel_W"
equation "d241 = tt_gearbox_H"
equation "d242 = tt_gearbox_W"
equation "d243 = -tt_gearbox_L"
equation "d247 = tt_can_D"
equation "d250 = tt_can_L"
equation "hammer_servo_L = 40.5 mm" comment "CONFIRMED: DS3218MG servo body length (incl. mount tabs), srituhobby.com listing"
equation "hammer_servo_W = 20 mm" comment "CONFIRMED: DS3218MG servo body width"
equation "hammer_servo_H = 40.5 mm" comment "CONFIRMED: DS3218MG servo body height"
equation "hammer_servo_horn_D = 25 mm" comment "MOCK: typical servo horn/spline envelope diameter"
equation "hammer_arm_L = 80 mm" comment "MOCK hammer arm length from pivot to head - NOT_FOR_MANUFACTURING, confirm reach vs chassis geometry"
equation "hammer_head_L = 30 mm" comment "MOCK hammer head length - NOT_FOR_MANUFACTURING"
equation "hammer_head_W = 20 mm" comment "MOCK hammer head width - NOT_FOR_MANUFACTURING"
equation "hammer_head_H = 15 mm" comment "MOCK hammer head height - NOT_FOR_MANUFACTURING"
equation "spinner_motor_D = 27.5 mm" comment "CONFIRMED: A2212 brushless motor can diameter (standard size)"
equation "spinner_motor_L = 30 mm" comment "CONFIRMED: A2212 brushless motor can length (standard size)"
equation "spinner_shaft_D = 4 mm" comment "DECIDED 2026-09-23: 4 mm weapon shaft (separate from the A2212 3.17 mm motor shaft; driven by 1:1 belt) to fit the 624 bearing"
equation "spinner_bearing_OD = 13 mm" comment "DECIDED 2026-09-23: 624 bearing, 4x13x5 mm, bore matches spinner_shaft_D"
equation "spinner_bar_L = 65 mm" comment "MOCK spinner weapon bar length (within spinner_gap_W envelope) - NOT_FOR_MANUFACTURING, needs structural review before fabrication"
equation "spinner_bar_W = 20 mm" comment "MOCK spinner weapon bar width - NOT_FOR_MANUFACTURING"
equation "spinner_bar_T = 6 mm" comment "MOCK spinner weapon bar thickness - NOT_FOR_MANUFACTURING"
equation "esc_L = 45 mm" comment "MOCK typical 30A BLHeli ESC envelope length"
equation "esc_W = 26 mm" comment "MOCK typical 30A ESC envelope width"
equation "esc_H = 8 mm" comment "MOCK typical 30A ESC envelope height"
equation "print_wall_t = 2 mm" comment "3D printed wall thickness placeholder (PETG typical)"
equation "d430 = battery_mock_L"
equation "d431 = battery_mock_W"
equation "d432 = battery_mock_H"
equation "d464 = base_t * 5"
equation "d466 = base_t * 5"
equation "d470 = ground_clearance + base_t"
equation "d473 = ground_clearance + base_t"
equation "d476 = ground_clearance + base_t"
equation "d485 = ground_clearance + base_t"
equation "d486 = -body_W / 2"
equation "d488 = wedge_depth"
equation "d489 = body_H - base_t"
equation "d490 = body_L / 2"
equation "d491 = ( body_W - spinner_gap_W ) / 2"
equation "d495 = ground_clearance + base_t"
equation "d496 = body_W / 2"
equation "d498 = wedge_depth"
equation "d499 = body_H - base_t"
equation "d500 = body_L / 2"
equation "d501 = -( body_W - spinner_gap_W ) / 2"
equation "d505 = ground_clearance + base_t"
equation "d508 = spinner_shaft_D"
equation "d513 = spinner_bearing_OD"
equation "d518 = spinner_bearing_OD"
equation "d528 = spinner_motor_D"
equation "m3_clear_d = 3.4 mm" comment "M3 clearance hole dia for CNC/laser-cut aluminum (tight fit)"
equation "m3_clear_d_fdm = 3.6 mm" comment "M3 clearance hole dia for FDM-printed parts (extra 0.2mm for print tolerance)"
equation "standoff_od = 6 mm" comment "M3 corner standoff outer diameter"
equation "standoff_bore_d = 3.2 mm" comment "Standoff through-bore for M3 screw (tap or use nut at one end)"
equation "tt_hole_spacing = 17.5 mm" comment "CONFIRMED: TT motor (all-metal gearbox variant) 2-hole M3 mount spacing, handsontec.com FAM1062 datasheet - verify against exact purchased unit"
equation "a2212_hole_x = 16 mm" comment "CONFIRMED: A2212 brushless motor rear mount hole spacing (short side), widely documented standard"
equation "a2212_hole_y = 19 mm" comment "CONFIRMED: A2212 brushless motor rear mount hole spacing (long side)"
equation "servo_flange_spacing = 49.5 mm" comment "CONFIRMED: standard servo flange mounting hole spacing (DS3218/MG996R-class), servodatabase.com"
equation "mount_plate_t = 3 mm" comment "Motor mounting bracket/plate thickness (aluminum)"
equation "d563 = standoff_od"
equation "d564 = standoff_bore_d"
equation "d565 = standoff_od"
equation "d566 = standoff_bore_d"
equation "d567 = standoff_od"
equation "d568 = standoff_bore_d"
equation "d569 = standoff_od"
equation "d570 = standoff_bore_d"
equation "d578 = side_t * 5"
equation "d580 = side_t * 5"
equation "d582 = tt_gearbox_L * 3"
equation "d584 = tt_gearbox_L * 3"
equation "d586 = spinner_motor_L * 3"
equation "d588 = base_t * 4"
equation "lip_h = 5 mm" comment "Battery holder side-lip height"
equation "strap_slot_w = 10 mm" comment "Battery strap slot width"
equation "strap_slot_l = 4 mm" comment "Battery strap slot length (thin slit)"
equation "pcb_standoff_h = 3 mm" comment "PCB standoff height (raises board off floor)"
equation "m2_5_clear_d_fdm = 2.9 mm" comment "M2.5 clearance hole for FDM-printed standoffs"
equation "d597 = battery_mock_L"
equation "d598 = battery_mock_W"
equation "d599 = print_wall_t"
equation "d601 = print_wall_t * 5"
equation "d605 = lip_h"
equation "d607 = lip_h"
equation "d639 = base_t * 6"
equation "d641 = base_t * 6"
equation "d643 = base_t * 6"
equation "d645 = base_t * 6"
equation "d657 = side_t * 6"
equation "d659 = side_t * 6"
equation "m2_clear_d = 2.2 mm" comment "M2 clearance hole for small electronics module mounting"
equation "roll_pin_d = 2 mm" comment "Roll pin diameter through shaft+bar - shock-resistant weapon fastening, stronger than friction set-screw alone"
equation "d695 = spinner_bar_W * 3"
named bodies: "Base_Plate_Al", "Left_Side_Plate_Al", "Right_Side_Plate_Al", "Left_Wheel", "Right_Wheel", "Top_Cover", "TT_Gearbox_L", "TT_Motor_Can_L", "TT_Gearbox_R", "TT_Motor_Can_R", "Battery_and_Tray", "Front_Wedge_L", "Front_Wedge_R", "Spinner_Shaft", "Left_Support", "Right_Support", "Spinner_Motor", "Standoff_1", "Standoff_2", "Standoff_3", "Standoff_4", "Battery_Holder", "Spinner_Motor_Cradle", "TT_Motor_Mount_L", "TT_Motor_Clamp_L", "TT_Motor_Mount_R", "TT_Motor_Clamp_R", "Batt_Post_1", "Batt_Post_2", "Batt_Post_3", "Batt_Post_4", "Disconnect_Post_1", "Disconnect_Post_2", "Rear_Panel", "Weapon_Pulley", "Motor_Pulley", "ESC_Tekko32", "Holder_ESC_Tekko32", "Rx_ER6", "Holder_Rx_ER6", "UBEC_5A", "Holder_UBEC_5A", "DRV8874_A", "Holder_DRV8874_A", "DRV8874_B", "Holder_DRV8874_B", "ESP32_DevKit", "ESP32_Module", "ESP32_Dupont_Keepout_A", "ESP32_Dupont_Keepout_B", "Holder_ESP32", "FingerTech_Switch_Adapter", "FingerTech_Mini_Switch_Envelope", "Beater_Rotor_Concept", "Beater_Sweep_Envelope"
